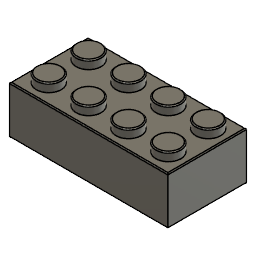
toy block (Autodesk Fusion 360 design; units mm, degrees)
part number: 2026-05-17-19-44-07-381
Autodesk Fusion 360 part; units mm, degrees
sketch "toy block" plane through (0, 0, 0) normal (0, 1, 0) x (1, 0, 0)
  line L0 (0, 0) -> (31.8, 0)
  line L1 (31.8, 0) -> (31.8, 15.8)
  line L2 (31.8, 15.8) -> (0, 15.8)
  line L3 (0, 15.8) -> (0, 0)
  dimension "d1" = 31.8
  dimension "d2" = 15.8
  constraint horizontal L0
  constraint vertical L1
  constraint horizontal L2
  constraint vertical L3
  constraint coincident L0.start L3.end
  measures "d1" distance of L0.start L0.end
  measures "d2" distance of L0.start L2.end
extrude "Extrude1" add sketch "toy block" along normal blind 9.6
sketch "Sketch2" plane through (0, 9.6, 0) normal (0, 1, 0) x (-1, 0, 0)
  line L0 (0, -15.8) -> (0, 0)
  line L1 (0, 0) -> (-31.8, 0)
  line L2 (-31.8, 0) -> (-31.8, -15.8)
  line L3 (-31.8, -15.8) -> (0, -15.8)
  circle A0 centre (-28, -3.9) radius 2.5
  dimension "d5" = 5
  dimension "d7" = 3.9
  dimension "d8" = 3.9
  measures "d5" diameter of A0
  measures "d7" distance of L1 A0.centre
  measures "d8" distance of L1 A0.centre
extrude "Extrude2" add sketch "Sketch2" along normal blind 1.7 contours A0
pattern_linear "R-Pattern1" count 4 spacing 8 along (-1, 0, 0) count 2 spacing 8 along (0, 0, -1) of "Extrude2"
shell "Shell1" thickness 1.49 removed faces 1 at (21.2, 0, -5.2667)
sketch "Sketch3" plane through (0, 8.11, 0) normal (0, -1, 0) x (1, 0, 0)
  line L0 (1.49, -1.49) -> (1.49, -14.31)
  line L1 (1.49, -14.31) -> (30.31, -14.31)
  line L2 (30.31, -14.31) -> (30.31, -1.49)
  line L3 (30.31, -1.49) -> (1.49, -1.49)
  circle A0 centre (28, -3.9) radius 1.01
  circle A1 centre (20, -3.9) radius 1.01
  circle A2 centre (12, -3.9) radius 1.01
  circle A3 centre (4, -3.9) radius 1.01
  circle A4 centre (28, -11.9) radius 1.01
  circle A5 centre (20, -11.9) radius 1.01
  circle A6 centre (12, -11.9) radius 1.01
  circle A7 centre (4, -11.9) radius 1.01
  line L4 (4, -3.9) -> (12, -11.9) construction
  circle A8 centre (8, -7.9) radius 3.15
  circle A9 centre (8, -7.9) radius 2.15
  dimension "d16" = 6.3
  dimension "d17" = -1
  constraint coincident A3.centre L4.start
  constraint coincident A6.centre L4.end
  constraint midpoint L4 A8.centre
  measures "d16" diameter of A8
extrude "Extrude3" add sketch "Sketch3" along normal blind 8.1 contours A8
pattern_linear "R-Pattern2" count 3 spacing 8 along (1, 0, 0) of "Extrude3"
fillet "Fillet1" radius 0.2 19 edges at (6.3308, 11.3, -4.804) (6.3308, 11.3, -12.804) (14.3308, 11.3, -12.804) (14.3308, 11.3, -4.804) (22.3308, 11.3, -12.804) (22.3308, 11.3, -4.804) (30.3308, 11.3, -4.804) (30.3308, 11.3, -12.804) (15.9, 9.6, -15.8) (0, 9.6, -7.9) (15.9, 9.6, 0) (13.0632, 0.01, -9.0391) (5.0632, 0.01, -9.0391) (5.0632, 8.11, -6.7609) (15.9, 0, 0) (31.8, 0, -7.9) (0, 0, -7.9) (15.9, 0, -15.8) (31.8, 9.6, -7.9)
